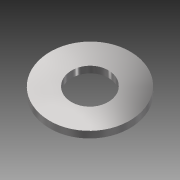
# Autodesk Inventor part: 275-1024
Saved by Autodesk Inventor 2016 (Build 200138000, 138)
## iProperties
Category: Structure
Company: Autodesk Inc.
Created: 2012-04-11
Part Number: 275-1024
Document SubType Name: Modeling
Designer: Autodesk Inc.
Density: 7.85 g/cm^3
Material: Steel
Catalog Web Link: http://www.vexrobotics.com/washers.html
Vendor: VEX
Mass: 0.359 g
Surface Area: 1.48008 cm^2
Volume: 0.0457324 cm^3
Appearance: Steel - Polished
Author: Autodesk Inc.
Autodesk Inventor part; units mm, degrees
ref_plane "YZ Plane" through (0, 0, 0) normal (1, 0, 0) x (0, 1, 0)
ref_plane "XZ Plane" through (0, 0, 0) normal (0, 1, 0) x (-1, 0, 0)
ref_plane "XY Plane" through (0, 0, 0) normal (0, 0, 1) x (1, 0, 0)
sketch "Sketch1" plane through (0, 0, 0) normal (0, 0, 1) x (1, 0, 0)
  circle A0 centre (-13.6107, 11.1425) radius 4.7625
  circle A1 centre (-13.6107, 11.1425) radius 2.1844
  dimension "d0" = 9.525
  dimension "d1" = 4.3688
  constraints: 2 centre point, 1 coincident
  measures "d0" diameter of A0
  measures "d1" diameter of A1
extrude "Extrusion1" add sketch "Sketch1" along normal blind 0.8128
body "Solid1"
